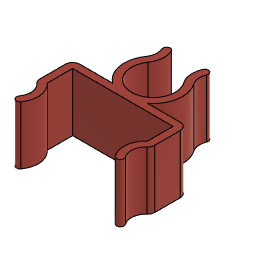
esc clip v2 (Autodesk Fusion 360 design; units mm, degrees)
Autodesk Fusion 360 part; units mm, degrees
note: some values were not read from the file. Chosen so that the rebuilt part matches the saved one: which face or edge a step refers to; which pieces of a blend or face edit are solid.
sketch "Sketch1" plane through (0, 0, 0) normal (0, 0, 1) x (1, 0, 0)
  line L0 (6.9, 2.5) -> (-6.9, 2.5)
  line L1 (-6.9, 2.5) -> (-6.9, -2.5)
  line L2 (-6.9, -2.5) -> (6.9, -2.5) construction
  line L3 (6.9, -2.5) -> (6.9, 2.5)
  line L4 (6.9, 2.5) -> (-6.9, -2.5) construction
  line L5 (-6.9, 2.5) -> (6.9, -2.5) construction
  line L6 (0, 6.7) -> (2.4575, 8.4207) construction
  line L7 (0, 0) -> (0, 16.1647)
  line L8 (0, 6.7) -> (-2.4575, 8.4207) construction
  arc A0 (-2.4575, 8.4207) -> (2.4575, 8.4207) centre (0, 6.7) ccw
  arc A1 (2.4575, 11.8622) -> (2.4575, 8.4207) centre (4.9149, 10.1415) ccw
  arc A2 (-2.4575, 8.4207) -> (-2.4575, 11.8622) centre (-4.9149, 10.1415) ccw
  arc A3 (-6.9, -5.4721) -> (-6.9, -1) centre (-8.9, -3.2361) ccw
  line L9 (-5.9, -5.3767) -> (-5.9, -1.8233) construction
  arc A4 (6.9, -1) -> (6.9, -5.4721) centre (8.9, -3.2361) ccw
  line L10 (-6.9, -1) -> (-6.9, 2.5)
  line L11 (6.9, -1) -> (6.9, 2.5)
  dimension "d1" = 13.8
  dimension "d2" = 5
  dimension "d4" = 6.7
  dimension "d5" = 35
  dimension "d6" = 3
  dimension "d7" = 3
  dimension "d9" = 3
  dimension "d10" = 1
  dimension "d11" = 3.5
  constraint horizontal L0
  constraint perpendicular L0 L1
  constraint parallel L0 L2
  constraint parallel L1 L3
  constraint coincident L4 L7.start
  constraint coincident L5 L7.start
  constraint coincident L7.start origin
  constraint perpendicular L0 L7
  constraint symmetric L6.start L7 L8.start
  constraint symmetric L6.end L7 L8.end
  constraint coincident L6.start L8.start
  constraint tangent A0 A1
  constraint vertical L6.end A1.start
  constraint symmetric L7 A1.start A2.end
  constraint symmetric L7 A1 A2
  constraint coincident L1 A3.end
  constraint perpendicular L2 L9
  constraint tangent A3 L9
  constraint vertical A3.end A3.start
  constraint symmetric L7 A3.end A4.start
  constraint symmetric L7 A3.start A4.end
  constraint symmetric L7 A3 A4
  constraint symmetric L0.end L7 L0.start
  measures "d1" distance of L1.end L2.end
  measures "d2" distance of L0.end L1.end
  measures "d4" vertical distance of L7.start L6.start
  measures "d5" angle of L0 L6
  measures "d6" radius of A0
  measures "d7" radius of A1
  measures "d9" radius of A3
  measures "d10" distance of L1 L9
  measures "d11" distance of L0.end A3.end
extrude "Extrude1" add sketch "Sketch1" along normal blind 8 thin wall 1 on the left open curves A2 A0 A1 A3 L10 L0 L11 A4
fillet "Fillet1" radius 0.5 2 edges at (3.2766, 11.2886, 4) (2.4575, 11.8622, 4)
fillet "Fillet1" radius 1.1472 2 edges at (-3.2766, 11.2886, 4) (-3.2766, 8.9943, 4)
fillet "Fillet1" radius 0.5 2 edges at (-2.4575, 11.8622, 4) (-3.2766, 11.2886, 4)
fillet "Fillet1" radius 1.62 2 edges at (7.5667, -4.7268, 4) (7.9, -1.504, 4)
fillet "Fillet1" radius 0.5 2 edges at (6.9, -5.4721, 4) (7.5667, -4.7268, 4)
fillet "Fillet1" radius 2.2361 2 edges at (6.9, -1, 4) (6.9, -5.4721, 4)
fillet "Fillet1" radius 0.5 2 edges at (-7.5667, -4.7268, 4) (-6.9, -5.4721, 4)
fillet "Fillet2" radius 1 4 edges at (7.9, 3.5, 4) (-7.9, 3.5, 4) (7.9, -1.504, 4) (-7.9, -1.504, 4)
equation "d1 = 13.7 mm + 0.1 mm"
equation "d2 = 4.9 mm + 0.1 mm"
equation "d3 = 6 mm"
equation "d4 = ( d3 + d2 ) / 2 + 1.2 mm"
equation "d7 = d6"
